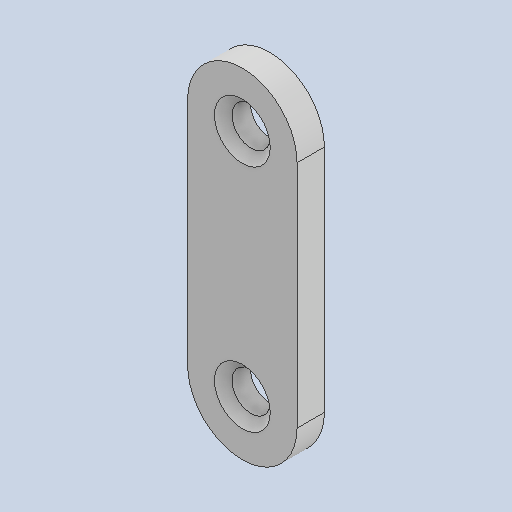
# Autodesk Inventor part: zaslepka
Saved by Autodesk Inventor 2023 (Build 270158000, 158)
## iProperties
Created: 2023-08-18
Part Number: zaslepka
Material: Ogólny
Document SubType Name: Modeling
Designer: Kamil
Density: 1 g/cm^3
Appearance: Domyślna
Author: Kamil
Autodesk Inventor part; units mm, degrees
ref_plane "YZ Plane" through (0, 0, 0) normal (1, 0, 0) x (0, 1, 0)
ref_plane "XZ Plane" through (0, 0, 0) normal (0, 1, 0) x (-1, 0, 0)
ref_plane "XY Plane" through (0, 0, 0) normal (0, 0, 1) x (1, 0, 0)
sketch "Szkic1" plane through (0, 0, 0) normal (0, 0, 1) x (1, 0, 0)
  line L0 (-17.5, 39.3937) -> (-17.5, -45.2473) projected
  line L1 (17.5, -26.5287) -> (-17.5, -45.2473) projected
  line L2 (17.5, 40.0799) -> (17.5, -26.5287) projected
  arc A0 (17.5, 40.0799) -> (16.7161, 41.0563) centre (16.5, 40.0799) ccw projected
  line L3 (3.9006, 43.8921) -> (16.7161, 41.0563) projected
  arc A1 (3.9006, 43.8921) -> (3.7868, 43.9105) centre (3.6845, 42.9157) ccw projected
  line L4 (3.7868, 43.9105) -> (-8.4909, 46.6272) projected
  arc A2 (-8.4909, 46.6272) -> (-17.5, 39.3937) centre (-10.0915, 39.3937) ccw projected
  line L5 (8.675, 4.2897) -> (8.675, -16.7103) projected
  arc A3 (-1.325, -16.7103) -> (8.675, -16.7103) centre (3.675, -16.7103) ccw projected
  line L6 (-1.325, -16.7103) -> (-1.325, 4.2897) projected
  arc A4 (8.675, 4.2897) -> (-1.325, 4.2897) centre (3.675, 4.2897) ccw projected
  point P0 (0, 0)
ref_plane "Płaszczyzna konstrukcyjna1" through (-1.325, -21.7103, -2.5) normal (0, 0, 1) x (1, 0, 0)
extrude "Wyciągnięcie proste1" add sketch "Szkic1" against normal up to surface (2.5 mm away) contours L5 A3 L6 A4
sketch "Szkic2" plane through (0, 0, 0) normal (0, 0, 1) x (1, 0, 0)
  circle A0 centre (3.675, 4.2897) radius 1.5 projected
  circle A1 centre (3.675, -16.7103) radius 1.5 projected
  arc A2 (8.675, 4.2897) -> (-1.325, 4.2897) centre (3.675, 4.2897) ccw projected
  point P0 (0, 0)
  constraints: 2 coincident
hole "Otwór1" at (3.675, 4.2897, 0) at (3.675, -16.7103, 0) direction (0, 0, -1) diameter 3.5 end through all countersink diameter 5.1 countersink angle 90
